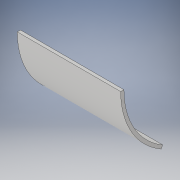
# Autodesk Inventor part: CollectorSweeperBacking
Saved by Autodesk Inventor 2019 (Build 230136000, 136)
## iProperties
Created: 2018-10-04
Part Number: CollectorSweeperBacking
Material: Generic
Document SubType Name: Modeling
Designer: User
Density: 1 g/cm^3
Appearance: Default
Author: User
Autodesk Inventor part; units mm, degrees
ref_plane "YZ Plane" through (0, 0, 0) normal (1, 0, 0) x (0, 1, 0)
ref_plane "XZ Plane" through (0, 0, 0) normal (0, 1, 0) x (-1, 0, 0)
ref_plane "XY Plane" through (0, 0, 0) normal (0, 0, 1) x (1, 0, 0)
sketch "Sketch1" plane through (0, 0, 0) normal (0, 1, 0) x (-1, 0, 0)
  line L0 (0, 0) -> (-23.9325, 0)
  line L1 (0, 76.2) -> (-101.6, 76.2)
  line L2 (-101.6, 76.2) -> (-101.6, 79.375)
  line L3 (-101.6, 79.375) -> (0, 79.375)
  line L4 (0, 79.375) -> (0, 76.2)
  dimension "d0" = 101.6
  dimension "d1" = 3.175
  dimension "d2" = 76.2
  constraints: 10 end point, 2 horizontal, 2 parallel, 1 perpendicular
  measures "d0" distance of L2.end L3.end
  measures "d1" distance of L1.end L2.end
  measures "d2" distance between parallel lines of L0 L1
revolve "Revolution1" add sketch "Sketch1" angle 60 about axis through (0, 0, 0) along (1, 0, 0)
body "Solid1"
